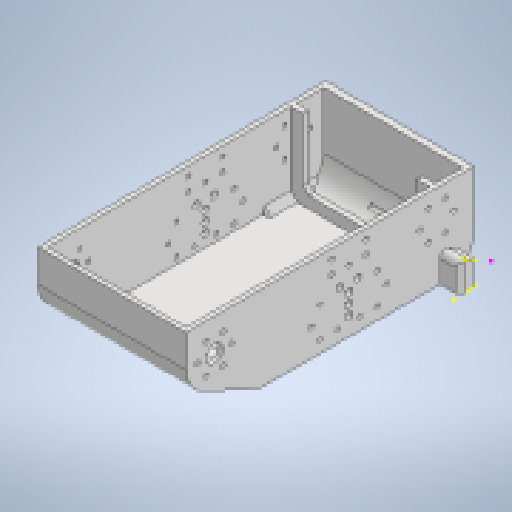
# Autodesk Inventor part: 车架
Saved by Autodesk Inventor 2025.1 (Build 291241000, 241)
## iProperties
Created: 2025-08-27
Part Number: 车架
Material: 常规
Document SubType Name: Modeling
Designer: Piw
Density: 1 g/cm^3
Appearance: 默认
Author: Piw
Autodesk Inventor part; units mm, degrees
ref_plane "YZ Plane" through (0, 0, 0) normal (1, 0, 0) x (0, 1, 0)
ref_plane "XZ Plane" through (0, 0, 0) normal (0, 1, 0) x (-1, 0, 0)
ref_plane "XY Plane" through (0, 0, 0) normal (0, 0, 1) x (1, 0, 0)
sketch "草图1" plane through (0, 0, 0) normal (0, 0, 1) x (1, 0, 0)
  line L0 (0, 5) -> (61, 5)
  line L1 (61, 5) -> (61, 75)
  line L2 (61, 75) -> (65, 75)
  line L3 (65, 75) -> (65, 0)
  line L4 (65, 0) -> (0, 0)
  line L5 (0, 34.2328) -> (0, -13.4923)
  line L6 (0, 5) -> (-61, 5)
  line L7 (-61, 5) -> (-61, 75)
  line L8 (-65, 75) -> (-65, 0)
  line L9 (-65, 0) -> (0, 0)
  line L10 (-61, 75) -> (-65, 75)
  dimension "d0" = 5
  dimension "d1" = 130
  dimension "d2" = 4
  dimension "d3" = 75
  constraints: 22 end point, 4 perpendicular, 4 symmetric about line, 2 vertical, 1 horizontal
  measures "d0" distance between parallel lines of L4 L0
  measures "d1" diameter of L3 L5
  measures "d2" distance between parallel lines of L3 L1
  measures "d3" distance between parallel lines of L4 L2
extrude "拉伸1" add sketch "草图1" along normal blind 138
sketch "草图2" plane through (65, 0, 0) normal (1, 0, 0) x (0, 0, -1)
  line L0 (-92.5, 24) -> (-57.5, 24) construction
  line L1 (0, 5) -> (-138, 5) projected
  circle A0 centre (-57.5, 24) radius 15.5 construction
  circle A1 centre (-92.5, 24) radius 15.5 construction
  circle A2 centre (-42, 24) radius 2.1
  circle A3 centre (-108, 24) radius 2.1
  line L2 (-138, 0) -> (-138, 75) projected
  circle A4 centre (-100.25, 10.5766) radius 2.1
  circle A5 centre (-84.75, 10.5766) radius 2.1
  circle A6 centre (-77, 24) radius 2.1
  circle A7 centre (-84.75, 37.4234) radius 2.1
  circle A8 centre (-100.25, 37.4234) radius 2.1
  circle A9 centre (-49.75, 37.4234) radius 2.1
  circle A10 centre (-65.25, 37.4234) radius 2.1
  circle A11 centre (-73, 24) radius 2.1
  circle A12 centre (-65.25, 10.5766) radius 2.1
  circle A13 centre (-49.75, 10.5766) radius 2.1
  point P0 (0, 0)
  dimension "d8" = 31
  dimension "d9" = 31
  dimension "d6" = 35
  dimension "d10" = 4.2
  dimension "d11" = 4.2
  dimension "d12" = 30
  dimension "d15" = 360
  dimension "d19" = 360
  dimension "d24" = 19
  constraints: 12 centre point, 2 coincident, 2 end point, 2 horizontal alignment, 2 point on line, 1 horizontal, 30 other
  measures "d6" distance of L0.start L0.end
  measures "d10" diameter of A2
  measures "d11" diameter of A3
  measures "d12" distance from line of L2 A3.centre
  measures "d24" distance between parallel lines of L1 L0
extrude "拉伸2" cut sketch "草图2" against normal blind 150 contours A2 | A3 | A4 | A5 | A8 | A9 | A12 | A13
sketch "草图3" plane through (65, 0, 0) normal (1, 0, 0) x (0, 0, -1)
  circle A0 centre (-75, 34) radius 3.25 projected
  circle A1 centre (-75, 25) radius 3.25 projected
  circle A2 centre (-75, 16) radius 3.25 projected
  circle A3 centre (-83, 41.2575) radius 3.25 projected
  circle A4 centre (-67, 41.2575) radius 3.25 projected
  point P0 (0, 0)
extrude "拉伸3" cut sketch "草图3" against normal blind 150
sketch "草图4" plane through (0, 0, 0) normal (0, 0, -1) x (-1, 0, 0)
  line L0 (-65, 0) -> (-65, 75) projected
  line L1 (65, 0) -> (-65, 0) projected
  line L2 (65, 75) -> (65, 0) projected
  line L3 (-65, 75) -> (-50, 75)
  line L4 (-50, 75) -> (-50, 15)
  line L5 (-50, 15) -> (50, 15)
  line L6 (50, 15) -> (50, 75)
  line L7 (50, 75) -> (65, 75)
  point P0 (0, 0)
  dimension "d27" = 15
  dimension "d28" = 15
  dimension "d29" = 15
  constraints: 10 end point, 4 perpendicular, 1 horizontal, 1 point on line
  measures "d27" distance between parallel lines of L1 L5
  measures "d28" distance between parallel lines of L2 L6
  measures "d29" distance between parallel lines of L4 L0
extrude "拉伸4" add sketch "草图4" along normal blind 5
sketch "草图5" plane through (0, 0, 0) normal (0, 0, 1) x (1, 0, 0)
  line L0 (61, 75) -> (61, 5) projected
  line L1 (50, 75) -> (61, 75) projected
  line L2 (50, 15) -> (50, 75) projected
  line L3 (-50, 15) -> (50, 15) projected
  line L4 (-50, 75) -> (-50, 15) projected
  line L5 (-61, 75) -> (-50, 75) projected
  line L6 (-61, 5) -> (-61, 75) projected
  line L7 (61, 5) -> (-61, 5) projected
  line L8 (61, 11) -> (55, 5)
  line L9 (0, 97.2027) -> (0, -45.2903)
  line L10 (-61, 11) -> (-55, 5)
  point P0 (0, 0)
  dimension "d32" = 45
  dimension "d33" = 6
  constraints: 6 end point, 2 point on line, 2 symmetric about line, 2 vertical
  measures "d32" angle of L0 L8
  measures "d33" horizontal distance of L8.end L8.start
extrude "拉伸5" add sketch "草图5" along normal blind 25 contours L0 L7 L8 | L7 L6 L10
chamfer "倒角1" distance 2 angle 45 2 edges at (58, 8, 25) (-58, 8, 25)
sketch "草图7" plane through (0, 0, 138) normal (0, 0, 1) x (1, 0, 0)
  line L0 (-65, 0) -> (65, 0) projected
  line L1 (65, 0) -> (65, 75) projected
  line L2 (65, 75) -> (61, 75) projected
  line L3 (61, 75) -> (61, 5) projected
  line L4 (61, 5) -> (-61, 5) projected
  line L5 (-61, 5) -> (-61, 75) projected
  line L6 (-61, 75) -> (-65, 75) projected
  line L7 (-65, 75) -> (-65, 0) projected
  point P0 (0, 0)
extrude "拉伸6" add sketch "草图7" along normal blind 15
sketch "草图8" plane through (-65, 0, -5) normal (-1, 0, 0) x (0, 0, 1)
  line L0 (158, 0) -> (158, 75) projected
  line L1 (158, 0) -> (223, 30.31)
  line L2 (223, 30.31) -> (223, 75)
  line L3 (223, 75) -> (158, 75)
  point P0 (5, 0)
  dimension "d41" = 65
  dimension "d42" = 65
  constraints: 6 end point, 1 parallel, 1 perpendicular
  measures "d41" distance between parallel lines of L0 L2
  measures "d42" angle of L0 L1
extrude "拉伸7" add sketch "草图8" against normal blind 4
sketch "草图10" plane through (-61, 11, 0) normal (1, 0, 0) x (0, 0, -1)
  line L0 (-218, 19.31) -> (-153, -11) projected
  line L1 (-218, 64) -> (-218, 19.31) projected
  line L2 (0, 64) -> (-218, 64) projected
  line L3 (-153, 64) -> (-153, -6) projected
  line L4 (-153, -6) -> (-214, 22.4448)
  line L5 (-214, 22.4448) -> (-214, 64)
  line L6 (-153, -6) -> (-153, -11) projected
  point P0 (0, -11)
  dimension "d46" = 4
  constraints: 4 end point, 2 parallel, 1 point on line
  measures "d46" distance between parallel lines of L1 L5
extrude "拉伸8" add sketch "草图10" along normal up to surface (122 mm away) contours L1 L2 L5 L4 L6 L0
sketch "草图11" plane through (61, 30.31, 218) normal (1, 0, 0) x (0, 0, -1)
  line L0 (65, -30.31) -> (65, 44.69) projected
  line L1 (218, 44.69) -> (4, 44.69) projected
  line L2 (4, 3.1348) -> (4, 44.69) projected
  line L3 (65, -25.31) -> (4, 3.1348) projected
  line L4 (0, 44.69) -> (0, 0) projected
  line L5 (0, 0) -> (65, -30.31) projected
  line L6 (4, 44.69) -> (0, 44.69) projected
  point P0 (218, -30.31)
extrude "拉伸9" add sketch "草图11" along normal blind 4
fillet "圆角1" radius 25 4 edges at (0, 30.31, 218) (0, 0, 153) (0, 5, 153) (0, 33.4448, 214)
sketch "草图12" plane through (65, 0, -5) normal (1, 0, 0) x (0, 0, -1)
  arc A0 (-223, 46.2368) -> (-208.5655, 23.5791) centre (-198, 46.2368) ccw projected
  circle A1 centre (-198, 46.2368) radius 15 construction
  circle A2 centre (-183, 46.2368) radius 2.1
  line L0 (-213, 46.2368) -> (-198, 46.2368) construction
  circle A3 centre (-190.5, 59.2271) radius 2.1
  circle A4 centre (-205.5, 59.2271) radius 2.1
  circle A5 centre (-213, 46.2368) radius 2.1
  circle A6 centre (-205.5, 33.2464) radius 2.1
  circle A7 centre (-190.5, 33.2464) radius 2.1
  circle A8 centre (-198, 46.2368) radius 7.5
  point P0 (-5, 0)
  dimension "d53" = 30
  dimension "d54" = 4.2
  dimension "d57" = 360
  dimension "d61" = 15
  constraints: 8 centre point, 2 coincident, 2 end point, 2 point on circle, 1 horizontal, 1 point on line, 13 other
  measures "d53" diameter of A1
  measures "d54" diameter of A2
  measures "d61" diameter of A8
extrude "拉伸10" cut sketch "草图12" against normal blind 150
sketch "草图13" plane through (-65, 0, -5) normal (-1, 0, 0) x (0, 0, 1)
  line L0 (65, 55) -> (95, 55) construction
  line L1 (95, 55) -> (95, 67) construction
  line L2 (95, 67) -> (65, 67) construction
  line L3 (65, 67) -> (65, 55) construction
  line L4 (65, 55) -> (95, 67) construction
  line L5 (95, 55) -> (65, 67) construction
  line L6 (0, 75) -> (223, 75) projected
  circle A0 centre (80, 34) radius 3.25 projected
  line L7 (80, 34) -> (80, 46.2012) construction
  circle A1 centre (65, 55) radius 2.1
  circle A2 centre (95, 55) radius 2.1
  circle A3 centre (80, 55) radius 2.1
  circle A4 centre (65, 67) radius 2.1
  circle A5 centre (95, 67) radius 2.1
  point P0 (5, 0)
  point P1 (80, 61)
  dimension "d62" = 8
  dimension "d63" = 30
  dimension "d64" = 20
  dimension "d65" = 4.2
  dimension "d66" = 4.2
  dimension "d67" = 4.2
  dimension "d68" = 4.2
  dimension "d69" = 4.2
  constraints: 14 end point, 5 centre point, 4 coincident, 3 midpoint, 2 parallel, 1 horizontal, 1 perpendicular, 1 point on line, 1 vertical
  measures "d62" distance between parallel lines of L6 L2
  measures "d63" distance between parallel lines of L1 L3
  measures "d64" distance between parallel lines of L6 L0
  measures "d65" diameter of A1
  measures "d66" diameter of A2
  measures "d67" diameter of A3
  measures "d68" diameter of A4
  measures "d69" diameter of A5
extrude "拉伸11" cut sketch "草图13" against normal blind 150 contours A1 | A2 | A3 | A4 | A5
sketch "草图14" plane through (0, 0, -5) normal (0, 0, -1) x (-1, 0, 0)
  line L0 (-61, 75) -> (-61, 11) projected
  line L1 (-55, 5) -> (55, 5) projected
  line L2 (-55, 5) -> (-61, 11) projected
  line L3 (61, 11) -> (61, 75) projected
  line L4 (61, 11) -> (55, 5) projected
  line L5 (65, 0) -> (65, 75) projected
  line L6 (-65, 0) -> (65, 0) projected
  line L7 (-65, 75) -> (-65, 0) projected
  line L8 (-50, 75) -> (-65, 75) projected
  line L9 (65, 75) -> (50, 75) projected
  point P0 (0, 0)
extrude "拉伸12" add sketch "草图14" along normal blind 30
sketch "草图15" plane through (-55, 5, -5) normal (0, 1, 0) x (1, 0, 0)
  line L0 (116, 0) -> (116, 30) projected
  line L1 (-6, 0) -> (-6, 30) projected
  line L2 (116, 30) -> (-6, 30)
  line L3 (-6, 30) -> (-6, 24)
  line L4 (-6, 24) -> (116, 24)
  line L5 (116, 24) -> (116, 30)
  point P0 (55, -5)
  dimension "d75" = 6
  constraints: 8 end point, 2 parallel, 1 horizontal, 1 perpendicular, 1 point on line
  measures "d75" distance between parallel lines of L2 L4
extrude "拉伸13" add sketch "草图15" along normal up to surface (70 mm away)
fillet "圆角2" radius 20 1 edges at (0, 5, -29)
fillet "圆角3" radius 25 1 edges at (0, 0, -35)
chamfer "倒角2" distance 5 angle 45 2 edges at (-50, 15, -2.5) (50, 15, -2.5)
sketch "草图16" plane through (65, 46.2368, 218) normal (1, 0, 0) x (0, 0, -1)
  circle A0 centre (220.5, 3.7632) radius 15 construction
  line L0 (228, -46.2368) -> (70.5424, -46.2368) projected
  line L1 (253, 28.7632) -> (253, -21.2368) projected
  circle A1 centre (235.5, 3.7632) radius 2.1
  line L2 (220.5, 3.7632) -> (205.5, 3.7632) construction
  circle A2 centre (228, 16.7536) radius 2.1
  circle A3 centre (213, 16.7536) radius 2.1
  circle A4 centre (205.5, 3.7632) radius 2.1
  circle A5 centre (213, -9.2271) radius 2.1
  circle A6 centre (228, -9.2271) radius 2.1
  circle A7 centre (220.5, 3.7632) radius 7.5
  point P0 (218, -46.2368)
  dimension "d83" = 30
  dimension "d84" = 50
  dimension "d85" = 32.5
  dimension "d86" = 4.2
  dimension "d89" = 360
  dimension "d91" = 15
  constraints: 8 centre point, 2 end point, 2 point on circle, 1 coincident, 1 horizontal, 1 point on line, 13 other
  measures "d83" diameter of A0
  measures "d84" distance from line of L0 L2.start
  measures "d85" distance from line of L1 L2.start
  measures "d86" diameter of A1
  measures "d91" diameter of A7
extrude "拉伸14" cut sketch "草图16" against normal blind 200 contours A1 | A2 | A3 | A4 | A5 | A6
sketch "草图17" plane through (65, 46.2368, 218) normal (1, 0, 0) x (0, 0, -1)
  line L0 (223.2626, -17.8554) -> (246.4689, -30.8806) projected
  line L1 (223.2626, -17.8554) -> (223.2626, -24.797)
  line L2 (223.2626, -24.797) -> (223.2626, -46.2368)
  arc A0 (228, -46.2368) -> (253, -21.2368) centre (228, -21.2368) ccw projected
  line L3 (228, -46.2368) -> (70.5424, -46.2368) projected
  line L4 (238.2626, -26.2746) -> (238.2626, -44.0332)
  point P0 (218, -46.2368)
  point P1 (250.1022, -32.9199)
  dimension "d96" = 15
  constraints: 6 end point, 2 point on line, 2 vertical, 1 point on circle
  measures "d96" distance between parallel lines of L2 L4
extrude "拉伸15" add sketch "草图17" along normal blind 18
sketch "草图18" plane through (83, 46.2368, 218) normal (1, 0, 0) x (0, 0, -1)
  arc A0 (228, -46.2368) -> (238.2626, -44.0332) centre (228, -21.2368) ccw projected
  line L0 (238.2626, -26.2746) -> (223.2626, -17.8554) projected
  point P0 (218, -46.2368)
  point P1 (250.1022, -32.9199)
sketch "草图19" plane through (-65, 46.2368, 218) normal (-1, 0, 0) x (0, 0, 1)
  line L0 (-223.2626, -17.8554) -> (-223.2626, -46.2368) projected
  line L1 (-223.2626, -46.2368) -> (-228, -46.2368) projected
  arc A0 (-238.2626, -44.0332) -> (-228, -46.2368) centre (-228, -21.2368) ccw projected
  line L2 (-238.2626, -44.0332) -> (-238.2626, -26.2746) projected
  line L3 (-238.2626, -26.2746) -> (-223.2626, -17.8554) projected
  point P0 (-218, -46.2368)
  point P1 (-238.2626, -44.0332)
extrude "拉伸16" add sketch "草图19" along normal blind 18
chamfer "倒角3" distance 4 angle 45 4 edges at (-83, 11.0828, -20.2626) (-83, 14.1907, -5.2626) (83, 11.0828, -20.2626) (83, 14.1907, -5.2626)
fillet "圆角4" radius 5 2 edges at (72, 28.3813, -5.2626) (-72, 28.3813, -5.2626)
sketch "草图22" plane through (65, 46.2368, 218) normal (1, 0, 0) x (0, 0, -1)
  arc A0 (228, -46.2368) -> (234.2626, -45.4396) centre (228, -21.2368) ccw projected
  line L0 (228, -46.2368) -> (247.1832, -46.2368)
  line L1 (247.1832, -46.2368) -> (252.1481, -27.7072)
  arc A1 (238.2626, -44.0332) -> (253, -21.2368) centre (228, -21.2368) ccw projected
  arc A2 (234.2626, -45.4396) -> (238.2626, -44.0332) centre (228, -21.2368) ccw projected
  point P0 (218, -46.2368)
  dimension "d114" = 105
  constraints: 4 end point, 2 tangent, 1 horizontal, 1 point on circle
  measures "d114" angle of L1 L0
extrude "拉伸19" add sketch "草图22" against normal up to surface (130 mm away)
sketch "草图23" plane through (65, 46.2368, 218) normal (1, 0, 0) x (0, 0, -1)
  circle A0 centre (243.3465, -41.2368) radius 1.9
  line L0 (247.1832, -46.2368) -> (252.1481, -27.7072) projected
  line L1 (228, -46.2368) -> (247.1832, -46.2368) projected
  point P0 (218, -46.2368)
  dimension "d117" = 3.8
  dimension "d118" = 5
  dimension "d119" = 5
  constraints: 1 centre point
  measures "d117" diameter of A0
  measures "d118" distance from line of L0 A0.centre
  measures "d119" distance from line of L1 A0.centre
extrude "拉伸20" cut sketch "草图23" against normal up to surface (130 mm away)
